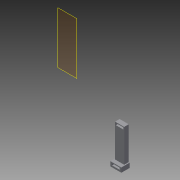
# Autodesk Inventor part: side piece
Saved by Autodesk Inventor 2015 (Build 190159000, 159)
## iProperties
Created: 2014-11-22
Part Number: side piece
Material: Generic
Document SubType Name: Modeling
Designer: jesse
Density: 1 g/cm^3
Appearance: Default
Author: jesse
Autodesk Inventor part; units mm, degrees
ref_plane "YZ Plane" through (0, 0, 0) normal (1, 0, 0) x (0, 1, 0)
ref_plane "XZ Plane" through (0, 0, 0) normal (0, 1, 0) x (-1, 0, 0)
ref_plane "XY Plane" through (0, 0, 0) normal (0, 0, 1) x (1, 0, 0)
ref_plane "Work Plane1" through (29.6407, 50.9726, 24.365) normal (0, 0, -1) x (-1, 0, 0)
sketch "Sketch1" plane through (29.6407, 50.9726, 24.365) normal (0, 0, -1) x (-1, 0, 0)
  line L0 (12.7, 3.175) -> (-12.7, 3.175) projected
  line L1 (-12.7, 3.175) -> (-12.7, -3.175) projected
  line L2 (-12.7, -3.175) -> (12.7, -3.175) projected
  line L3 (12.7, -3.175) -> (12.7, 3.175) projected
  line L4 (-12.7, -113.4117) -> (12.7, -113.4117) projected
  line L5 (12.7, -113.4117) -> (12.7, -107.0617) projected
  line L6 (12.7, -107.0617) -> (-12.7, -107.0617) projected
  line L7 (-12.7, -107.0617) -> (-12.7, -113.4117) projected
  line L8 (-15.24, -5.715) -> (-15.24, 5.715)
  line L9 (-15.24, 5.715) -> (15.24, 5.715)
  line L10 (15.24, 5.715) -> (15.24, -5.715)
  line L11 (15.24, -96.743) -> (15.24, -115.9518)
  line L12 (15.24, -115.9518) -> (-15.24, -115.9518)
  line L13 (-15.24, -115.9518) -> (-15.24, -96.743)
  line L14 (-15.24, -5.715) -> (-15.24, -96.743)
  line L15 (15.24, -5.715) -> (15.24, -98.1393)
  point P0 (29.6407, -50.9726)
  constraints: 16 end point, 1 point on line, 4 other
extrude "Extrusion1" add sketch "Sketch1" against normal blind 12.7
sketch "Sketch2" plane through (29.6407, 50.9726, 24.365) normal (0, 0, -1) x (-1, 0, 0)
  line L0 (15.24, -115.9518) -> (15.24, 5.715) projected
  line L1 (-15.24, -115.9518) -> (15.24, -115.9518) projected
  line L2 (-15.24, 5.715) -> (-15.24, -115.9518) projected
  line L3 (15.24, 5.715) -> (-15.24, 5.715) projected
  point P0 (29.6407, -50.9726)
extrude "Extrusion2" add sketch "Sketch2" along normal blind 2.54
sketch "Sketch3" plane through (29.6407, 50.9726, 37.065) normal (0, 0, 1) x (1, 0, 0)
  line L0 (-12.7, -113.4117) -> (-12.7, -107.0617) projected
  line L1 (-12.7, -107.0617) -> (12.7, -107.0617) projected
  line L2 (12.7, -107.0617) -> (12.7, -113.4117) projected
  line L3 (12.7, -113.4117) -> (-12.7, -113.4117) projected
  line L4 (12.7, 3.175) -> (12.7, -3.175) construction
  line L5 (12.7, -3.175) -> (-12.7, -3.175) construction
  line L6 (-12.7, -3.175) -> (-12.7, 3.175) construction
  line L7 (-12.7, 3.175) -> (12.7, 3.175) construction
  line L8 (-15.24, 5.715) -> (-15.24, -115.9518) construction
  line L9 (-15.24, -115.9518) -> (15.24, -115.9518) construction
  line L10 (15.24, -115.9518) -> (15.24, 5.715) construction
  line L11 (15.24, 5.715) -> (-15.24, 5.715) construction
  line L12 (18.415, -119.1268) -> (-18.415, -119.1268)
  line L13 (-18.415, -119.1268) -> (-18.415, -103.8867)
  line L14 (-18.415, -103.8867) -> (18.415, -103.8867)
  line L15 (18.415, -103.8867) -> (18.415, -119.1268)
  line L16 (18.415, -119.1268) -> (-18.415, -103.8867) construction
  line L17 (-18.415, -119.1268) -> (18.415, -103.8867) construction
  point P0 (-29.6407, -50.9726)
  point P1 (0, -111.5068)
  dimension "d6" = 3.175
  dimension "d9" = 3.175
  dimension "d10" = 3.175
  dimension "d11" = 3.175
  constraints: 12 end point, 2 midpoint, 2 parallel, 1 horizontal, 1 perpendicular
  measures "d6" distance between parallel lines of L12 L9
  measures "d9" distance between parallel lines of L15 L10
  measures "d10" distance between parallel lines of L13 L8
  measures "d11" distance between parallel lines of L1 L14
extrude "Extrusion3" add sketch "Sketch3" against normal up to surface (15.24 mm away)
sketch "Sketch4" plane through (29.6407, 50.9726, 37.065) normal (0, 0, 1) x (1, 0, 0)
  line L0 (-12.7, -113.4117) -> (-12.7, -107.0617) projected
  line L1 (-12.7, -107.0617) -> (12.7, -107.0617) projected
  line L2 (12.7, -107.0617) -> (12.7, -113.4117) projected
  line L3 (12.7, -113.4117) -> (-12.7, -113.4117) projected
  line L4 (-18.415, -103.8867) -> (-15.24, -103.8867) projected
  line L5 (-18.415, -119.1268) -> (-18.415, -103.8867) projected
  line L6 (18.415, -119.1268) -> (-18.415, -119.1268) projected
  line L7 (18.415, -103.8867) -> (18.415, -119.1268) projected
  line L8 (15.24, -103.8867) -> (18.415, -103.8867) projected
  line L9 (15.24, -103.8867) -> (15.24, 5.715) projected
  line L10 (15.24, 5.715) -> (-15.24, 5.715) projected
  line L11 (-15.24, 5.715) -> (-15.24, -103.8867) projected
  line L12 (12.7, 3.175) -> (12.7, -3.175) projected
  line L13 (12.7, -3.175) -> (-12.7, -3.175) projected
  line L14 (-12.7, -3.175) -> (-12.7, 3.175) projected
  line L15 (-12.7, 3.175) -> (12.7, 3.175) projected
  line L16 (15.24, -103.8867) -> (-15.24, -103.8867)
  point P0 (-29.6407, -50.9726)
  constraints: 2 end point, 1 horizontal
extrude "Extrusion4" add sketch "Sketch4" along normal blind 12.7 contours L4 L16 L8 L7 L6 L5
body "Solid1"
